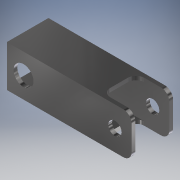
# Autodesk Inventor part: bracket2
Saved by Autodesk Inventor 2018.2 (Build 222227000, 227)
## iProperties
Created: 2018-03-19
Part Number: bracket2
Material: 鉄、可鍛鉄
Document SubType Name: Modeling
Designer: ku_sk
Density: 7.15 g/cm^3
Appearance: 半つや出し
Author: ku_sk
Autodesk Inventor part; units mm, degrees
ref_plane "YZ Plane" through (0, 0, 0) normal (1, 0, 0) x (0, 1, 0)
ref_plane "XZ Plane" through (0, 0, 0) normal (0, 1, 0) x (-1, 0, 0)
ref_plane "XY Plane" through (0, 0, 0) normal (0, 0, 1) x (1, 0, 0)
sketch "スケッチ1" plane through (0, 0, 0) normal (1, 0, 0) x (0, 1, 0)
  line L0 (-12.5, 12.5) -> (12.5, 12.5)
  line L1 (12.5, 12.5) -> (12.5, -12.5)
  line L2 (12.5, -12.5) -> (-12.5, -12.5)
  line L3 (-12.5, -12.5) -> (-12.5, 12.5)
  line L4 (-12.5, 12.5) -> (12.5, -12.5) construction
  line L5 (12.5, 12.5) -> (-12.5, -12.5) construction
  point P0 (0, 0)
  dimension "d0" = 25
  dimension "d1" = 25
  constraints: 12 end point, 2 midpoint, 2 parallel, 1 horizontal, 1 perpendicular
  measures "d0" distance of L0.start L0.end
  measures "d1" distance of L0.end L1.end
extrude "押し出し1" add sketch "スケッチ1" along normal blind 75
sketch "スケッチ2" plane through (0, 12.5, 12.5) normal (0, 1, 0) x (1, 0, 0)
  circle A0 centre (10, 12.5) radius 6
  line L0 (0, 0) -> (0, 25) projected
  line L1 (0, 0) -> (75, 0) projected
  point P0 (0, 12.5)
  dimension "d4" = 12
  dimension "d5" = 10
  dimension "d6" = 12.5
  constraints: 1 centre point
  measures "d4" diameter of A0
  measures "d5" distance from line of L0 A0.centre
  measures "d6" distance from line of A0.centre L1
extrude "押し出し2" cut sketch "スケッチ2" against normal through all
sketch "スケッチ3" plane through (0, 12.5, 12.5) normal (0, 1, 0) x (1, 0, 0)
  circle A0 centre (65, 12.5) radius 4
  line L0 (75, 25) -> (75, 0) projected
  line L1 (0, 25) -> (75, 25) projected
  point P0 (0, 12.5)
  dimension "d9" = 10
  dimension "d10" = 8
  dimension "d11" = 12.5
  constraints: 1 centre point
  measures "d9" distance from line of L0 A0.centre
  measures "d10" diameter of A0
  measures "d11" distance from line of L1 A0.centre
extrude "押し出し3" cut sketch "スケッチ3" against normal through all
sketch "スケッチ4" plane through (75, 0, 0) normal (1, 0, 0) x (0, 0, -1)
  line L0 (-10.2, -10.2) -> (10.2, -10.2)
  line L1 (10.2, -10.2) -> (10.2, 10.2)
  line L2 (10.2, 10.2) -> (-10.2, 10.2)
  line L3 (-10.2, 10.2) -> (-10.2, -10.2)
  line L4 (-10.2, -10.2) -> (10.2, 10.2) construction
  line L5 (10.2, -10.2) -> (-10.2, 10.2) construction
  line L6 (-12.5, 12.5) -> (-12.5, -12.5) projected
  line L7 (12.5, 12.5) -> (-12.5, 12.5) projected
  point P0 (0, 0)
  dimension "d14" = 2.3
  dimension "d15" = 2.3
  constraints: 12 end point, 2 midpoint, 2 parallel, 1 horizontal, 1 perpendicular
  measures "d14" distance between parallel lines of L6 L3
  measures "d15" distance between parallel lines of L7 L2
extrude "押し出し4" cut sketch "スケッチ4" against normal through all
sketch "スケッチ5" plane through (0, -12.5, -12.5) normal (0, 0, -1) x (-1, 0, 0)
  line L0 (-75, 2.3) -> (-75, 22.7) projected
  line L1 (-75, 22.7) -> (-55, 22.7)
  line L2 (-55, 22.7) -> (-55, 2.3)
  line L3 (-55, 2.3) -> (-75, 2.3)
  line L4 (-75, 2.3) -> (-75, 22.7)
  line L5 (-75, 2.3) -> (0, 2.3) projected
  point P0 (0, 12.5)
  dimension "d18" = 20
  constraints: 8 end point, 2 parallel, 1 collinear, 1 horizontal, 1 perpendicular
  measures "d18" distance of L2.end L3.end
extrude "押し出し5" cut sketch "スケッチ5" against normal through all
fillet "フィレット1" radius 5 8 edges at (55, 10.2, 11.35) (55, 10.2, -11.35) (75, 11.35, -12.5) (75, 11.35, 12.5) (75, -11.35, -12.5) (75, -11.35, 12.5) (55, -10.2, 11.35) (55, -10.2, -11.35)
equation "\"d1\" = d0"
